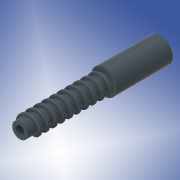
# Autodesk Inventor part: BA014
Saved by Autodesk Inventor 2017 (Build 210142000, 142)
## iProperties
Created: 2017-06-28
Part Number: BA014
Material: ABS Plastic
Document SubType Name: Modeling
Designer: zallen
Density: 1.06 g/cm^3
Appearance: CR Dark Blue
Author: zallen
Autodesk Inventor part; units mm, degrees
ref_plane "YZ Plane" through (0, 0, 0) normal (1, 0, 0) x (0, 1, 0)
ref_plane "XZ Plane" through (0, 0, 0) normal (0, 1, 0) x (-1, 0, 0)
ref_plane "XY Plane" through (0, 0, 0) normal (0, 0, 1) x (1, 0, 0)
sketch "Sketch5" plane through (0, 0, 0) normal (0, 0, 1) x (1, 0, 0)
  circle A0 centre (0, 0) radius 5.5
  dimension "d13" = 11
  constraints: 1 centre point, 1 coincident
  measures "d13" diameter of A0
extrude "Extrusion2" add sketch "Sketch5" along normal blind 100
sketch "Sketch7" plane through (0, 0, 100) normal (0, 0, 1) x (1, 0, 0)
  circle A0 centre (0, 0) radius 3
  dimension "d29" = 6
  constraints: 1 centre point, 1 coincident
  measures "d29" diameter of A0
extrude "Extrusion3" cut sketch "Sketch7" against normal through all
sketch "Sketch6" plane through (0, 0, 0) normal (0, 1, 0) x (-1, 0, 0)
  line L0 (5.5, 100) -> (-5.5, 100) projected
  line L1 (5.5, 0) -> (5.5, 100) projected
  line L2 (5.5, 96) -> (7.5, 96)
  line L3 (7.5, 96) -> (7.5, 94)
  line L4 (7.5, 94) -> (5.5, 94)
  line L5 (5.5, 96) -> (5.5, 94)
  line L6 (0, 100) -> (0, 0)
  point P0 (7.5, 95)
  dimension "d17" = 2
  dimension "d18" = 2
  dimension "d20" = 4
  constraints: 10 end point, 3 perpendicular, 2 coincident, 2 midpoint, 2 vertical, 1 point on line
  measures "d17" distance of L2.start L2.end
  measures "d18" distance of L2.end L3.end
  measures "d20" distance between parallel lines of L0 L2
coil "Coil2" sketch "Sketch6" operation add axis through (0, 0, 100) along (0, 0, -1) pitch 5.6 turns 10 hand right
chamfer "Chamfer1" distance 0.5 angle 45 40 edges at (0, 7.5, 94.6) (0, 7.5, 89) (0, -7.5, 91.8) (0, -7.5, 86.2) (0, 7.5, 83.4) (0, -7.5, 80.6) (0, 7.5, 77.8) (0, -7.5, 75) (0, 7.5, 72.2) (0, -7.5, 41.4) (0, -7.5, 69.4) (0, 7.5, 66.6) (0, 7.5, 44.2) (0, -7.5, 47) (0, -7.5, 63.8) (0, 7.5, 61) (0, 7.5, 49.8) (0, -7.5, 52.6) (0, -7.5, 58.2) (0, 7.5, 55.4) (0, 7.5, 92.6) (0, -7.5, 89.8) (0, 7.5, 87) (0, -7.5, 84.2) (0, 7.5, 81.4) (0, -7.5, 78.6) (0, 7.5, 75.8) (0, -7.5, 39.4) (0, -7.5, 45) (0, 7.5, 42.2) (0, -7.5, 73) (0, 7.5, 70.2) (0, -7.5, 50.6) (0, 7.5, 47.8) (0, -7.5, 67.4) (0, 7.5, 64.6) (0, -7.5, 56.2) (0, 7.5, 53.4) (0, -7.5, 61.8) (0, 7.5, 59)
sketch "Sketch9" plane through (0, 0, 0) normal (0, 0, -1) x (-1, 0, 0)
  circle A0 centre (0, 0) radius 3 projected
  circle A1 centre (0, 0) radius 5.5 projected
  circle A2 centre (0, 0) radius 9
  dimension "d39" = 18
  constraints: 1 centre point, 1 coincident
  measures "d39" diameter of A2
extrude "Extrusion5" add sketch "Sketch9" against normal blind 40 contours A2
sketch "Sketch8" plane through (0, 0, 0) normal (1, 0, 0) x (0, 1, 0)
  circle A0 centre (0, 8) radius 1.5
  point P0 (0, 0)
  dimension "d35" = 3
  dimension "d36" = 8
  constraints: 1 centre point, 1 vertical alignment
  measures "d35" diameter of A0
  measures "d36" distance of point (0, 0) A0.centre
extrude "Extrusion4" cut sketch "Sketch8" against normal through all
body "Solid2"
